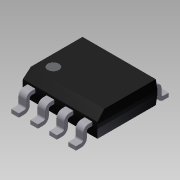
# Autodesk Inventor part: SOIC-08
Saved by Autodesk Inventor 2011 (Build 150239000, 239)
## iProperties
Created: 2010-11-20
Part Number: SOIC-08
Document SubType Name: Modeling
Designer: abbath
Density: 1 g/cm^3
Author: abbath
Autodesk Inventor part; units mm, degrees
ref_plane "YZ Plane" through (0, 0, 0) normal (1, 0, 0) x (0, 1, 0)
sketch "Эскиз1" plane through (0, 0, 0) normal (0, 0, 1) x (1, 0, 0)
  line L0 (-2.5, 2) -> (2.5, 2)
  line L1 (2.5, 2) -> (2.5, -2)
  line L2 (2.5, -2) -> (-2.5, -2)
  line L3 (-2.5, -2) -> (-2.5, 2)
  point P0 (0, 0)
  dimension "d0" = 2.5
  dimension "d1" = 2
  dimension "d2" = 5
  dimension "d3" = 4
  constraints: 8 end point, 2 parallel, 1 horizontal, 1 perpendicular
  measures "d0" distance from line of L3 point (0, 0)
  measures "d1" distance from line of L0 point (0, 0)
  measures "d2" distance between parallel lines of L1 L3
  measures "d3" distance between parallel lines of L2 L0
extrude "Выдавливание1" add sketch "Эскиз1" along normal blind 1.75
sketch "Эскиз4" plane through (2.5, -2, 0) normal (1, 0, 0) x (0, 0, -1)
  line L0 (-1.75, 4) -> (-1.75, 0) projected
  line L1 (0, 0) -> (-1.75, 0) projected
  line L2 (0, 4) -> (0, 0) projected
  line L3 (0, 4) -> (-1.75, 4) projected
  line L4 (-1.125, 0) -> (-1.125, 4)
  line L5 (-0.875, 0) -> (-0.875, 4)
  line L6 (-1.125, 0) -> (-1.262, 0.012)
  line L7 (-1.125, 4) -> (-1.75, 3.9453)
  line L8 (-0.25, 3.9453) -> (-0.25, 0.0547)
  line L9 (-0.25, 0.0547) -> (-0.875, 0)
  line L10 (-0.875, 4) -> (-0.25, 3.9453)
  line L11 (-1.75, 0.5) -> (-1.262, 0.012)
  point P0 (0, 2)
  dimension "d18" = 0.625
  dimension "d19" = 0.25
  dimension "d20" = 0.25
  dimension "d21" = 0.625
  dimension "d22" = 5
  dimension "d23" = 5
  dimension "d24" = 45
  dimension "d25" = 0.5
  constraints: 16 end point, 4 parallel, 4 point on line, 2 midpoint, 1 perpendicular
  measures "d18" distance between parallel lines of L4 L0
  measures "d19" distance between parallel lines of L2 L8
  measures "d20" distance between parallel lines of L5 L4
  measures "d21" distance between parallel lines of L8 L5
  measures "d22" angle of L1 L6
  measures "d23" angle of L3 L7
  measures "d24" angle of L11 L0
  measures "d25" distance from line of L11.start L1
extrude "Выдавливание4" cut sketch "Эскиз4" against normal through all contours L3 L7 L0 | L11 L6 L1 L0 | L3 L2 L1 L9 L8 L10
sketch "Эскиз5" plane through (-2.5, -2, 0.875) normal (0, -1, 0) x (1, 0, 0)
  line L0 (5, 0) -> (5, 0.25) projected
  line L1 (0, 0.387) -> (0, 0.875) projected
  line L2 (5, 0.387) -> (0, 0.387) projected
  line L3 (5, 0.875) -> (5, 0.387) projected
  line L4 (0, 0.875) -> (5, 0.875) projected
  line L5 (0, 0.25) -> (0, 0.387) projected
  line L6 (5, 0.25) -> (0, 0.25) projected
  line L7 (5, 0.387) -> (5, 0.25) projected
  line L8 (5, 0.387) -> (0, 0.387) projected
  line L9 (0, -0.625) -> (0, 0) projected
  line L10 (5, -0.625) -> (0, -0.625) projected
  line L11 (5, 0) -> (5, -0.625) projected
  line L12 (0, 0) -> (5, 0) projected
  line L13 (0, 0.25) -> (0.0547, 0.875)
  line L14 (5, 0.25) -> (4.9453, 0.875)
  line L15 (5, 0) -> (4.9453, -0.625)
  line L16 (0, 0) -> (0.0547, -0.625)
  line L17 (4.9453, 0.875) -> (5, 0.875)
  line L18 (5, 0.875) -> (5, 0.25)
  line L19 (0.0547, 0.875) -> (0, 0.875)
  line L20 (0, 0.875) -> (0, 0.25)
  point P0 (2.5, -0.875)
  dimension "d28" = 5
  dimension "d29" = 5
  constraints: 16 end point, 4 point on line, 3 perpendicular, 2 parallel, 1 collinear
  measures "d28" angle of L1 L13
  measures "d29" angle of L3 L14
extrude "Выдавливание5" cut sketch "Эскиз5" against normal through all contours L14 L2 L7 | L11 L10 L15 | L16 L10 L9 | L5 L2 L13 | L2 L14 L4 L3 | L1 L4 L13 L2
ref_plane "РабПлоскость1" through (-1.905, -2, 0.875) normal (-1, 0, 0) x (0, 0, 1)
sketch "Эскиз6" plane through (-1.905, -2, 0.875) normal (-1, 0, 0) x (0, 0, 1)
  line L0 (0.875, 0.5) -> (0.387, 0.012) projected
  line L1 (0.875, 3.9453) -> (0.875, 0.5) projected
  line L2 (0.25, 4) -> (0.875, 3.9453) projected
  line L3 (0.25, 0) -> (0.25, 4) projected
  line L4 (0.387, 0.012) -> (0.25, 0) projected
  line L5 (0, 4) -> (0, 0) projected
  line L6 (0, 0) -> (0.25, 0) projected
  line L7 (0.25, 0) -> (0.25, 4) projected
  line L8 (0, 4) -> (0.25, 4) projected
  line L9 (-0.625, 3.9453) -> (0, 4) projected
  line L10 (-0.625, 0.0547) -> (-0.625, 3.9453) projected
  line L11 (0, 0) -> (-0.625, 0.0547) projected
  line L12 (0, 4) -> (0, 0) projected
  line L13 (-0.875, 2) -> (1.3511, 2) construction
  line L14 (0.25, 0) -> (0.25, -0.2417)
  line L15 (0, 0) -> (0, -0.2417)
  line L16 (0.25, 0) -> (0, 0)
  line L17 (-0.625, -1.1) -> (-0.875, -1.1)
  line L18 (-0.875, -1.1) -> (-0.875, -0.7417)
  line L19 (-0.625, -0.7417) -> (-0.625, -1.1)
  line L20 (-0.125, -0.3667) -> (-0.5, -0.3667)
  line L21 (-0.125, -0.6167) -> (-0.5, -0.6167)
  arc A0 (-0.125, -0.3667) -> (0, -0.2417) centre (-0.125, -0.2417) ccw
  arc A1 (-0.5, -0.6167) -> (-0.625, -0.7417) centre (-0.5, -0.7417) ccw
  arc A2 (-0.125, -0.6167) -> (0.25, -0.2417) centre (-0.125, -0.2417) ccw
  arc A3 (-0.5, -0.3667) -> (-0.875, -0.7417) centre (-0.5, -0.7417) ccw
  dimension "d42" = 0.25
  dimension "d43" = 3.1
  dimension "d44" = 0.25
  dimension "d45" = 0.25
  dimension "d46" = 1.1
  dimension "d47" = 0.7333
  dimension "d48" = 0.25
  dimension "d49" = 0.25
  dimension "d50" = 0.25
  constraints: 19 end point, 8 point on circle, 6 collinear, 6 perpendicular, 6 tangent, 4 centre point, 3 parallel, 2 coincident, 1 point on line
  measures "d42" distance between parallel lines of L15 L14
  measures "d43" distance between parallel lines of L17 L13
  measures "d44" distance between parallel lines of L18 L10
  measures "d45" distance between parallel lines of L18 L19
  measures "d46" distance between parallel lines of L17 L6
  measures "d47" distance between parallel lines of L17 L20
  measures "d48" distance between parallel lines of L21 L20
  measures "d49" diameter of A0
  measures "d50" diameter of A1
extrude "Выдавливание6" add sketch "Эскиз6" along normal mid plane 0.51 contours L14 A2 L21 A1 L19 L17 L18 A3 L20 A0 L15 L6
ref_plane "РабПлоскость2" through (2.5, 0, 0.875) normal (0, -1, 0) x (1, 0, 0)
mirror "Зеркальное отражение1" about plane through (2.5, 0, 0.875) normal (0, -1, 0) of "Выдавливание6"
pattern_linear "Прямоуг.массив1" count 4 spacing 1.27 along (1, 0, 0) of "Выдавливание6", "Зеркальное отражение1"
sketch "Эскиз7" plane through (0, 0, 1.75) normal (0, 0, 1) x (1, 0, 0)
  line L0 (-2.4453, 1.9453) -> (-2.4453, -1.5) projected
  line L1 (-2.4453, -1.5) -> (2.4453, -1.5) projected
  circle A0 centre (-1.6953, -0.75) radius 0.375
  point P0 (0, 0)
  dimension "d57" = 0.75
  dimension "d58" = 0.75
  dimension "d59" = 0.75
  constraints: 1 centre point
  measures "d57" diameter of A0
  measures "d58" distance from line of L0 A0.centre
  measures "d59" distance from line of L1 A0.centre
extrude "Выдавливание7" cut sketch "Эскиз7" against normal blind 0.01
equation "\"d0\" = 0.5 * d2"
equation "\"d1\" = 0.5 * d3"
equation "\"d18\" = d21"
equation "\"d45\" = d42"
equation "\"d47\" = 0.666667 * d46"
equation "\"d48\" = d44"
equation "\"d49\" = d44"
equation "\"d50\" = d51"
equation "\"d51\" = 0.25"
